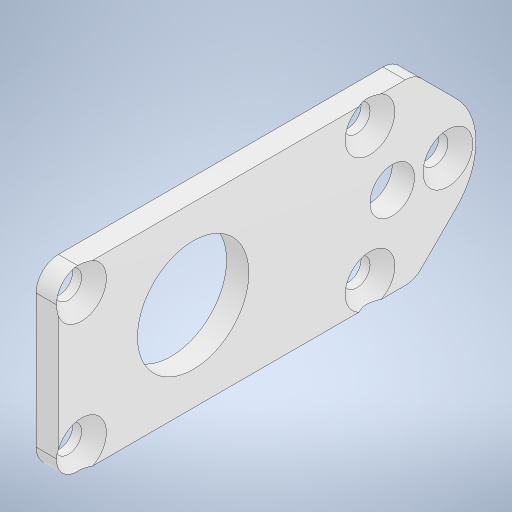
# Autodesk Inventor part: Face PLate
Saved by Autodesk Inventor 2023.2 (Build 272271000, 271)
## iProperties
Created: 2023-07-16
Part Number: Face PLate
Material: UHMW, White
Document SubType Name: Modeling
Designer: Nathan Cai
Density: 0.94 g/cm^3
Appearance: Smooth - White
Mass: 3.50691 g
Surface Area: 32.5028 cm^2
Volume: 3.73075 cm^3
Author: Nathan Cai
Autodesk Inventor part; units mm, degrees
ref_plane "YZ Plane" through (0, 0, 0) normal (1, 0, 0) x (0, 1, 0)
ref_plane "XZ Plane" through (0, 0, 0) normal (0, 1, 0) x (-1, 0, 0)
ref_plane "XY Plane" through (0, 0, 0) normal (0, 0, 1) x (1, 0, 0)
sketch "Sketch1" plane through (0, 0, 0) normal (1, 0, 0) x (0, 1, 0)
  line L0 (-12.7, 25.4) -> (12.7, 25.4)
  line L1 (12.7, 25.4) -> (12.7, -25.4)
  line L2 (12.7, -25.4) -> (-12.7, -25.4) construction
  line L3 (-12.7, -25.4) -> (-12.7, 25.4)
  line L4 (-12.7, 25.4) -> (12.7, -25.4) construction
  line L5 (12.7, 25.4) -> (-12.7, -25.4) construction
  line L6 (0, 25.4) -> (0, -25.4) construction
  circle A0 centre (0, -22.225) radius 3.175
  line L7 (-3.175, -15.875) -> (3.175, -15.875) construction
  line L8 (3.175, -15.875) -> (3.175, -34.925) construction
  line L9 (3.175, -34.925) -> (-3.175, -34.925)
  line L10 (-3.175, -34.925) -> (-3.175, -15.875) construction
  line L11 (-3.175, -15.875) -> (3.175, -34.925) construction
  line L12 (3.175, -15.875) -> (-3.175, -34.925) construction
  line L13 (12.7, -25.4) -> (3.175, -34.925)
  line L14 (-3.175, -34.925) -> (-12.7, -25.4)
  circle A1 centre (0, 6.175) radius 7.9375
  point P0 (0, 0)
  dimension "d0" = 25.4
  dimension "d1" = 50.8
  dimension "d2" = 6.35
  dimension "d4" = 6.35
  dimension "d5" = 9.525
  dimension "d6" = 15.875
  dimension "d7" = 28.4
  constraints: 30 end point, 6 midpoint, 4 parallel, 2 centre point, 2 horizontal, 2 perpendicular, 2 point on line, 1 tangent
  measures "d0" distance of L1.end L2.end
  measures "d1" distance of L0.end L1.end
  measures "d2" diameter of A0
  measures "d4" distance of L8.end L9.end
  measures "d5" distance between parallel lines of L2 L9
  measures "d6" diameter of A1
  measures "d7" distance of A0.centre A1.centre
extrude "Extrusion1" add sketch "Sketch1" along normal blind 3.175
fillet "Fillet1" radius 9.525 2 edges at (1.5875, 3.175, -34.925) (1.5875, -3.175, -34.925)
fillet "Fillet2" radius 3.175 4 edges at (1.5875, 12.7, 25.4) (1.5875, -12.7, 25.4) (1.5875, 12.7, -25.4) (1.5875, -12.7, -25.4)
sketch "Sketch2" plane through (3.175, 0, 0) normal (1, 0, 0) x (0, 0, -1)
  point P0 (19.05, 9.525)
  point P1 (30.1625, 0)
  point P2 (19.05, -9.525)
  point P3 (-22.098, 9.525)
  point P4 (-22.098, -9.525)
hole "Hole1" at (3.175, 9.525, -19.05) at (3.175, 0, -30.1625) at (3.175, -9.525, -19.05) at (3.175, 9.525, 22.098) at (3.175, -9.525, 22.098) direction (-1, 0, 0) diameter 3.7973 end through all countersink diameter 7.0866 countersink angle 82
body "Solid1"
